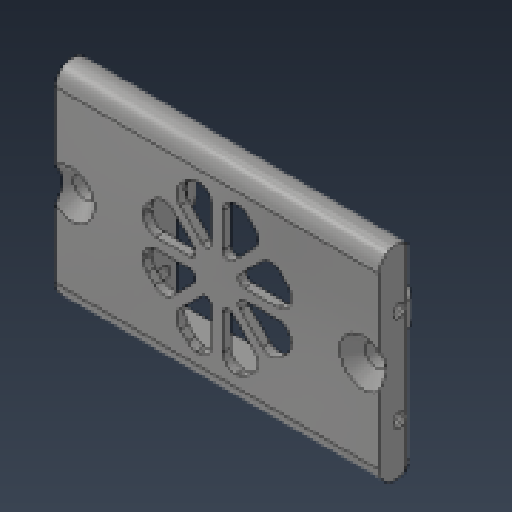
# Autodesk Inventor part: PCBs_Holder
Saved by Autodesk Inventor 2026.2 (Build 302298010, 298A)
## iProperties
Created: 2026-04-14
Part Number: PCBs_Holder
Material: Nylon 6/6
Document SubType Name: Modeling
Designer: szymo
Density: 1.13 g/cm^3
Appearance: Nylon 6(1)
Mass: 2.82412 g
Surface Area: 26.3379 cm^2
Volume: 2.49922 cm^3
Author: szymo
Autodesk Inventor part; units mm, degrees
ref_plane "YZ Plane" through (0, 0, 0) normal (1, 0, 0) x (0, 1, 0)
ref_plane "XZ Plane" through (0, 0, 0) normal (0, 1, 0) x (-1, 0, 0)
ref_plane "XY Plane" through (0, 0, 0) normal (0, 0, 1) x (1, 0, 0)
sketch "Sketch1" plane through (0, 0, 0) normal (0, 0, 1) x (1, 0, 0)
  line L0 (19.2, 23.1) -> (-19.2, 23.1)
  line L1 (-19.2, 23.1) -> (-19.2, 47.2371)
  line L2 (-19.2, 47.2371) -> (19.2, 47.2371)
  line L3 (19.2, 47.2371) -> (19.2, 23.1)
  line L4 (15.2, 33.6685) -> (10.2, 33.6685)
  line L5 (10.2, 33.6685) -> (10.2, 36.6685)
  line L6 (10.2, 36.6685) -> (15.2, 36.6685)
  line L7 (15.2, 36.6685) -> (15.2, 33.6685)
  line L8 (-15.2, 33.6685) -> (-10.2, 33.6685)
  line L9 (-10.2, 33.6685) -> (-10.2, 36.6685)
  line L10 (-10.2, 36.6685) -> (-15.2, 36.6685)
  line L11 (-15.2, 36.6685) -> (-15.2, 33.6685)
  line L12 (8.75, 43.9185) -> (-8.75, 43.9185)
  line L13 (-8.75, 43.9185) -> (-8.75, 26.4185)
  line L14 (-8.75, 26.4185) -> (8.75, 26.4185)
  line L15 (8.75, 26.4185) -> (8.75, 43.9185)
  line L16 (-19.2, 25.795) -> (-15.4, 25.795) projected
  line L17 (-19.2, 45.542) -> (-15.4, 45.542) projected
  line L18 (-19.2, 25.795) -> (-19.2, 45.542) projected
  circle A0 centre (-17.3, 35.1685) radius 1.0065 projected
  line L19 (19.2, 25.795) -> (15.4, 25.795) projected
  line L20 (19.2, 25.795) -> (19.2, 45.542) projected
  line L21 (19.2, 45.542) -> (15.4, 45.542) projected
  circle A1 centre (17.3, 35.1685) radius 1.0065 projected
  line L22 (15.4, 25.795) -> (15.4, 45.542) projected
  line L23 (-15.4, 25.795) -> (-15.4, 45.542) projected
  point P0 (0, 0)
  point P1 (-17.3, 35.1685)
  point P2 (17.3, 35.1685)
  point P3 (-15.2, 23.1)
  point P4 (-15.2, 47.2371)
  point P5 (15.2, 23.1)
  point P6 (15.2, 47.2371)
  point P7 (19.2, 23.1)
  point P8 (19.2, 47.2371)
  point P9 (-19.2, 47.2371)
  point P10 (-19.2, 23.1)
  dimension "d4" = 10.5685
  dimension "d5" = 10.5685
  dimension "d6" = 10.5685
  dimension "d7" = 10.5685
  dimension "d10" = 3
  dimension "d11" = 3
  dimension "d12" = 5
  dimension "d13" = 5
  dimension "d45" = 17.5
  dimension "d46" = 17.5
  dimension "d47" = 3.3185
  dimension "d48" = 3.3185
  dimension "d49" = 10.45
  dimension "d50" = 10.45
  dimension "d83" = 12.0685
  dimension "d84" = 12.0685
  dimension "d85" = 12.0685
  dimension "d86" = 12.0685
  dimension "d110" = 0.2
  dimension "d111" = 0.2
  constraints: 32 end point, 8 parallel, 4 horizontal, 4 perpendicular, 2 point on line
  measures "d4" distance between parallel lines of L0 L4
  measures "d5" distance between parallel lines of L0 L8
  measures "d6" distance between parallel lines of L2 L6
  measures "d7" distance between parallel lines of L2 L10
  measures "d10" distance between parallel lines of L6 L4
  measures "d11" distance between parallel lines of L10 L8
  measures "d12" distance between parallel lines of L7 L5
  measures "d13" distance between parallel lines of L9 L11
  measures "d45" distance between parallel lines of L14 L12
  measures "d46" distance between parallel lines of L13 L15
  measures "d47" distance between parallel lines of L2 L12
  measures "d48" distance between parallel lines of L0 L14
  measures "d49" distance between parallel lines of L3 L15
  measures "d50" distance between parallel lines of L1 L13
  measures "d83" distance from line of L2 point (17.3, 35.169)
  measures "d84" distance from line of L0 point (17.3, 35.169)
  measures "d85" distance from line of point (-17.3, 35.169) L2
  measures "d86" distance from line of L0 point (-17.3, 35.169)
  measures "d110" distance between parallel lines of L23 L11
  measures "d111" distance between parallel lines of L22 L7
extrude "Extrusion3" add sketch "Sketch1" against normal blind 4 contours L0 L1 L16 L23 L17 L2 L3 L21 L22 L19 | L19 L22 L21 L3 | L1 L17 L23 L16 | L4 L5 L6 L7 | L11 L10 L9 L8 | A0 | A1
extrude "Extrusion4" add sketch "Sketch1" against normal blind 9.2 contours L4 L5 L6 L7 | L11 L10 L9 L8
hole "Hole2" at (-17.3, 35.1685, 0) at (17.3, 35.1685, 0) direction (0, 0, -1) diameter 2.5 end through all countersink diameter 5.5 countersink angle 90 clearance for "Countersunk Flat Head Screw ISO 2009/7046" size "M2.5" standard "ISO"
fillet "Fillet6" radius 2 4 edges at (0, 47.2371, -4) (0, 23.1, -4) (0, 23.1, 0) (0, 47.2371, 0)
sketch "Sketch3" plane through (10.2, 33.6685, -4) normal (0, -1, 0) x (1, 0, 0)
  line L0 (0, 0) -> (0, -5.2) projected
  line L1 (5, -5.2) -> (0, -5.2) projected
  line L2 (5, 0) -> (5, -5.2) projected
  line L3 (-25.4, 0) -> (-25.4, -5.2) projected
  line L4 (-20.4, -5.2) -> (-25.4, -5.2) projected
  line L5 (-20.4, 0) -> (-20.4, -5.2) projected
  line L6 (-25.4, 0) -> (-20.4, 0) projected
  line L7 (0, 0) -> (5, 0) projected
  line L8 (5, -0.2) -> (-25.4, -0.2)
  line L9 (5, -0.2) -> (0, -5.2)
  line L10 (5, -5.2) -> (0, -0.2)
  line L11 (-20.4, -5.2) -> (-25.4, -0.2)
  line L12 (-20.4, -0.2) -> (-25.4, -5.2)
  point P0 (2.5, -2.7)
  point P1 (-22.9, -2.7)
  dimension "d109" = 0.2
  constraints: 10 end point, 6 point on line, 3 midpoint, 1 parallel, 1 perpendicular
  measures "d109" distance between parallel lines of L8 L7
hole "Hole3" at (12.7, 33.6685, -6.7) at (-12.7, 33.6685, -6.7) direction (0, 1, 0) diameter 2.5 end through all
sketch "Sketch6" plane through (19.2, 37.1566, 0) normal (1, 0, 0) x (0, 0, -1)
  circle A0 centre (2.4, 3.1124) radius 0.7 projected
  circle A1 centre (2.4, -8.1314) radius 0.7 projected
  point P0 (0, -37.1566)
  point P1 (2.9912, -7.7566)
  point P2 (1.8088, -7.7566)
hole "Hole5" at (19.2, 40.2691, -2.4) at (19.2, 29.0252, -2.4) direction (-1, 0, 0) diameter 1.567 depth 15 thread size "M2x0.4" class "6H" standard "ISO Metric profile"
sketch "Sketch7" plane through (-19.2, 23.1, 0) normal (-1, 0, 0) x (0, 0, 1)
  circle A0 centre (-2.4, 6.9913) radius 0.7 projected
  circle A1 centre (-2.4, 18.0712) radius 0.7 projected
  point P0 (0, -23.1)
hole "Hole6" at (-19.2, 30.0913, -2.4) at (-19.2, 41.1712, -2.4) direction (1, 0, 0) diameter 1.567 depth 15 thread size "M2x0.4" class "6H" standard "ISO Metric profile"
sketch "Sketch8" plane through (10.2, 36.6685, -4) normal (0, 1, 0) x (1, 0, 0)
  line L0 (-20.4, 0) -> (-25.4, 0) projected
  line L1 (-20.4, 0) -> (-20.4, 5.2) projected
  line L2 (-25.4, 5.2) -> (-20.4, 5.2) projected
  line L3 (-25.4, 0) -> (-25.4, 5.2) projected
  line L4 (5, 0) -> (0, 0) projected
  line L5 (5, 0) -> (5, 5.2) projected
  line L6 (0, 5.2) -> (5, 5.2) projected
  line L7 (0, 0) -> (0, 5.2) projected
  circle A0 centre (2.5, 2.7) radius 2.5
  line L8 (0, 2.7) -> (0, 0)
  line L9 (5, 2.7) -> (5, 0)
  line L10 (9, 0) -> (-29.4, 0) projected
  circle A1 centre (-22.9, 2.7) radius 2.5
  line L11 (-25.4, 2.7) -> (-25.4, 0)
  line L12 (-20.4, 2.7) -> (-20.4, 0)
  circle A2 centre (-22.9, 2.7) radius 1.25 projected
  circle A3 centre (2.5, 2.7) radius 1.25 projected
  point P0 (-10.2, -4)
  point P1 (-13.45, 0)
  point P2 (2.5, 5.2)
  point P3 (-22.9, 5.2)
  point P4 (-20.4, 2.7)
  point P5 (-25.4, 2.7)
  point P6 (5, 2.7)
  point P7 (0, 2.7)
  point P8 (1, 4.2)
  point P9 (1.3126, 0)
  point P10 (3.6874, 0)
  point P11 (-24.0874, 0)
  point P12 (-21.7126, 0)
  point P13 (-24.4, 4.2)
  dimension "d103" = 5
  dimension "d104" = 5
  constraints: 8 end point, 4 point on circle, 4 point on line, 4 tangent, 3 perpendicular, 2 centre point, 2 coincident, 1 collinear
  measures "d103" diameter of A0
  measures "d104" diameter of A1
extrude "Extrusion6" cut sketch "Sketch8" against normal up to surface (3 mm away) contours A1 L2 L1 | L3 L2 A1 | A0 L6 L5 | L7 L6 A0
sketch "Sketch9" plane through (0, 0, 0) normal (0, 0, 1) x (1, 0, 0)
  line L0 (-8.75, 43.9185) -> (8.75, 43.9185) projected
  line L1 (-8.75, 26.4185) -> (-8.75, 43.9185) projected
  line L2 (8.75, 43.9185) -> (8.75, 26.4185) projected
  line L3 (8.75, 26.4185) -> (-8.75, 26.4185) projected
  line L4 (3.0931, 43.9185) -> (8.75, 38.2617)
  line L5 (-8.75, 43.9185) -> (8.75, 26.4185) construction
  line L6 (-8.75, 26.4185) -> (8.75, 43.9185) construction
  line L7 (-8.75, 38.2617) -> (-3.0931, 43.9185)
  line L8 (-3.0931, 26.4185) -> (-8.75, 32.0754)
  line L9 (8.75, 32.0754) -> (3.0931, 26.4185)
  line L10 (-0.625, 43.9185) -> (-0.625, 26.4185)
  line L11 (0.625, 26.4185) -> (0.625, 43.9185)
  line L12 (-8.75, 35.7935) -> (8.75, 35.7935)
  line L13 (-8.75, 34.5435) -> (8.75, 34.5435)
  line L14 (-5.4796, 41.5321) -> (-0.625, 36.6774)
  line L15 (0.625, 36.6774) -> (5.4796, 41.5321)
  line L16 (6.3635, 40.6482) -> (1.5089, 35.7935)
  line L17 (1.5089, 34.5435) -> (6.3635, 29.6889)
  line L18 (5.4796, 28.805) -> (0.625, 33.6597)
  line L19 (-6.3635, 29.6889) -> (-1.5089, 34.5435)
  line L20 (-6.3635, 40.6482) -> (-1.5089, 35.7935)
  line L21 (-5.4796, 28.805) -> (-0.625, 33.6597)
  point P0 (0, 0)
  point P1 (0, 35.1685)
  point P2 (0, 35.1685)
  point P3 (-8.75, 38.2617)
  point P4 (-3.0931, 26.4185)
  point P5 (3.0931, 26.4185)
  point P6 (8.75, 32.0754)
  point P7 (-3.0931, 43.9185)
  point P8 (-0.625, 35.7935)
  point P9 (-0.625, 34.5435)
  point P10 (-8.75, 32.0754)
  dimension "d112" = 45
  dimension "d113" = 4
  dimension "d116" = 360
  dimension "d118" = 0.625
  dimension "d119" = 0.625
  dimension "d120" = 0.625
  dimension "d121" = 0.625
  dimension "d122" = 0.625
  dimension "d124" = 0.625
  dimension "d125" = 0.625
  dimension "d126" = 0.625
  dimension "d127" = 0.625
  dimension "d128" = 0.625
  dimension "d129" = 0.625
  dimension "d130" = 0.625
  constraints: 36 end point, 26 point on line, 7 perpendicular, 5 parallel, 2 midpoint, 13 other
  measures "d112" angle of L0 L4
  measures "d113" distance from line of L0.end L4
  measures "d118" distance from line of L13 point (0, 35.169)
  measures "d119" distance from line of L12 point (0, 35.169)
  measures "d120" distance from line of L10 point (0, 35.169)
  measures "d121" distance from line of L11 point (0, 35.169)
  measures "d122" distance between parallel lines of L5 L20
  measures "d124" distance between parallel lines of L5 L14
  measures "d125" distance between parallel lines of L6 L15
  measures "d126" distance between parallel lines of L16 L6
  measures "d127" distance between parallel lines of L5 L17
  measures "d128" distance between parallel lines of L5 L18
  measures "d129" distance between parallel lines of L6 L21
  measures "d130" distance between parallel lines of L19 L6
extrude "Extrusion7" add sketch "Sketch9" against normal blind 1 contours L0 L7 L1 | L0 L11 L12 L10 | L14 L10 L12 L20 L7 | L12 L10 L13 L1 | L0 L2 L4 | L15 L4 L16 L12 L11 | L12 L11 L13 L10 | L8 L3 L1 | L13 L10 L21 L8 L19 | L12 L2 L13 L11 | L13 L11 L3 L10 | L13 L17 L9 L18 L11 | L9 L2 L3
fillet "Fillet8" radius 1 2 edges at (-19.2, 35.1685, -4) (19.2, 35.1685, -4)
fillet "Fillet7" radius 1.5 24 edges at (-3.0931, 43.9185, -0.5) (-0.625, 43.9185, -0.5) (0.625, 43.9185, -0.5) (3.0931, 43.9185, -0.5) (5.4796, 41.5321, -0.5) (6.3635, 40.6482, -0.5) (8.75, 38.2617, -0.5) (8.75, 35.7935, -0.5) (8.75, 34.5435, -0.5) (8.75, 32.0754, -0.5) (6.3635, 29.6889, -0.5) (5.4796, 28.805, -0.5) (3.0931, 26.4185, -0.5) (0.625, 26.4185, -0.5) (-0.625, 26.4185, -0.5) (-3.0931, 26.4185, -0.5) (-5.4796, 28.805, -0.5) (-6.3635, 29.6889, -0.5) (-8.75, 32.0754, -0.5) (-8.75, 34.5435, -0.5) (-8.75, 35.7935, -0.5) (-8.75, 38.2617, -0.5) (-6.3635, 40.6482, -0.5) (-5.4796, 41.5321, -0.5)
fillet "Fillet9" radius 0.7 8 edges at (-1.5089, 35.7935, -0.5) (-1.5089, 34.5435, -0.5) (-0.625, 33.6597, -0.5) (0.625, 33.6597, -0.5) (1.5089, 34.5435, -0.5) (1.5089, 35.7935, -0.5) (0.625, 36.6774, -0.5) (-0.625, 36.6774, -0.5)
equation "\"d4\" = d6"
equation "\"d5\" = d7"
equation "\"d11\" = d10"
equation "\"d13\" = d12"
equation "\"d47\" = d48"
equation "\"d49\" = d50"
body "Solid2"
